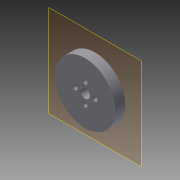
# Autodesk Inventor part: smallGearMag01
Saved by Autodesk Inventor 2013 (Build 170138000, 138)
## iProperties
Created: 2013-03-04
Part Number: smallGearMag01
Material: Generic
Document SubType Name: Modeling
Designer: Nano
Density: 1 g/cm^3
Author: Nano
Autodesk Inventor part; units mm, degrees
ref_plane "YZ Plane" through (0, 0, 0) normal (1, 0, 0) x (0, 1, 0)
ref_plane "XZ Plane" through (0, 0, 0) normal (0, 1, 0) x (-1, 0, 0)
ref_plane "XY Plane" through (0, 0, 0) normal (0, 0, 1) x (1, 0, 0)
ref_plane "Work Plane1" through (0, 0, 0) normal (0, 0, 1) x (1, 0, 0)
sketch "Sketch1" plane through (0, 0, 0) normal (0, 0, 1) x (1, 0, 0)
  circle A0 centre (0, 0) radius 3.0861 projected
  circle A1 centre (6.35, 0) radius 1.5875 projected
  circle A2 centre (0, 6.35) radius 1.5875 projected
  circle A3 centre (-6.35, 0) radius 1.5875 projected
  circle A4 centre (0, -6.35) radius 1.5875 projected
  circle A5 centre (0, 0) radius 19.2656
  point P0 (0, 0)
  constraints: 1 centre point
extrude "Extrusion1" add sketch "Sketch1" along normal blind 6.35
body "Solid1"
